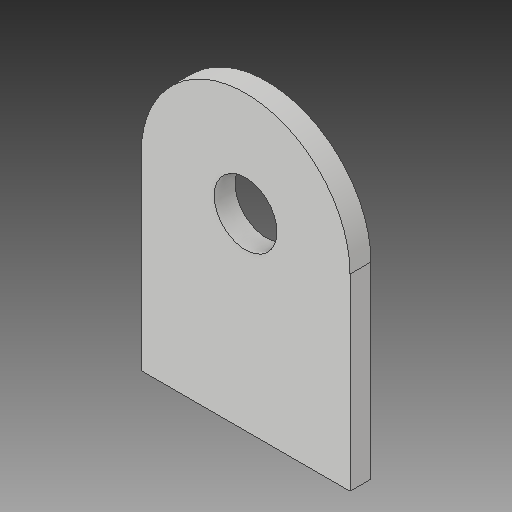
# Autodesk Inventor part: podporka
Saved by Autodesk Inventor 2019 (Build 230136000, 136)
## iProperties
Created: 2019-12-14
Part Number: podporka
Material: Ogólny
Document SubType Name: Modeling
Designer: Karolina
Density: 1 g/cm^3
Appearance: Domyślna
Author: Karolina
Autodesk Inventor part; units mm, degrees
ref_plane "YZ Plane" through (0, 0, 0) normal (1, 0, 0) x (0, 1, 0)
ref_plane "XZ Plane" through (0, 0, 0) normal (0, 1, 0) x (-1, 0, 0)
ref_plane "XY Plane" through (0, 0, 0) normal (0, 0, 1) x (1, 0, 0)
sketch "Szkic1" plane through (0, 0, 0) normal (0, 0, 1) x (1, 0, 0)
  line L0 (-10, 14) -> (0, 14)
  line L1 (0, 14) -> (0, 0)
  line L2 (0, 0) -> (-10, 0)
  line L3 (-10, 0) -> (-10, 14)
  point P0 (-5, 9)
  dimension "d0" = 10
  dimension "d5" = 5
  dimension "d6" = 5
  dimension "d7" = 9
  constraints: 8 end point, 2 parallel, 1 horizontal, 1 perpendicular
  measures "d0" distance of L0.start L0.end
  measures "d5" distance from line of L0 point (-5, 9)
  measures "d6" horizontal distance of L0.start point (-5, 9)
  measures "d7" distance from line of L2 point (-5, 9)
extrude "Wyciągnięcie proste1" add sketch "Szkic1" along normal mid plane 1
fillet "Zaokrąglenie1" radius 5 2 edges at (0, 14, 0) (-10, 14, 0)
hole "Otwór1" at (-5, 9, 0) direction (0, 0, 1) diameter 3 end through all both
